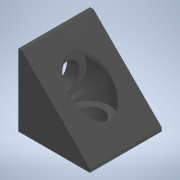
# Autodesk Inventor part: Black Angle Corner Connector
Saved by Autodesk Inventor 2022 (Build 260153000, 153)
## iProperties
Created: 2016-04-10
Part Number: Black Angle Corner Connector
Material: Generic
Document SubType Name: Modeling
Designer: Ben
Density: 1 g/cm^3
Appearance: Default
VLDS_Profile: Default Part
VLDS_TimeStamp: 2022-03-14
VLDS_FailCnt: 4
VLDS_AcceptCnt: 0
Author: Ben
Autodesk Inventor part; units mm, degrees
ref_plane "YZ Plane" through (0, 0, 0) normal (1, 0, 0) x (0, 1, 0)
ref_plane "XZ Plane" through (0, 0, 0) normal (0, 1, 0) x (-1, 0, 0)
ref_plane "XY Plane" through (0, 0, 0) normal (0, 0, 1) x (1, 0, 0)
sketch "Sketch1" plane through (0, 0, 0) normal (0, 0, 1) x (1, 0, 0)
  line L0 (0, 0) -> (20, 0)
  line L1 (20, 0) -> (20, 1)
  line L2 (20, 1) -> (1, 20)
  line L3 (1, 20) -> (0, 20)
  line L4 (0, 20) -> (0, 0)
  dimension "d0" = 135
  dimension "d1" = 20
  dimension "d2" = 20
  dimension "d3" = 1
  constraints: 10 end point, 2 parallel, 1 horizontal, 1 perpendicular
  measures "d0" angle of L2 L1
  measures "d1" distance of L3.end L0.start
  measures "d2" distance of L0.start L0.end
  measures "d3" distance of L0.end L1.end
extrude "Extrusion1" add sketch "Sketch1" along normal mid plane 20
sketch "Sketch2" plane through (0, 0, 10) normal (0, -1, 0) x (1, 0, 0)
  circle A0 centre (10, -10) radius 3.57
  point P0 (0, -10)
  dimension "d6" = 7.14
  constraints: 1 centre point
  measures "d6" diameter of A0
extrude "Extrusion2" cut sketch "Sketch2" against normal blind 3.5
sketch "Sketch3" plane through (10, 3.5, 0) normal (0, -1, 0) x (1, 0, 0)
  circle A0 centre (0, 0) radius 3.57 projected
  circle A1 centre (0, 0) radius 5.5
  point P0 (-10, 0)
  dimension "d9" = 11
  constraints: 1 centre point, 1 coincident
  measures "d9" diameter of A1
extrude "Extrusion3" cut sketch "Sketch3" against normal up to next contours A0 | A1
sketch "Sketch4" plane through (0, 0, 10) normal (-1, 0, 0) x (0, 0, 1)
  circle A0 centre (-10, 10) radius 3.57
  point P0 (-10, 0)
  dimension "d12" = 7.14
  constraints: 1 centre point
  measures "d12" diameter of A0
extrude "Extrusion4" cut sketch "Sketch4" against normal blind 3.5
sketch "Sketch5" plane through (3.5, 10, 0) normal (-1, 0, 0) x (0, 0, 1)
  circle A0 centre (0, 0) radius 3.57 projected
  circle A1 centre (0, 0) radius 5.5
  point P0 (0, -10)
  dimension "d15" = 11
  constraints: 1 centre point, 1 coincident
  measures "d15" diameter of A1
extrude "Extrusion5" cut sketch "Sketch5" against normal up to next contours A0 | A1
body "Solid1"
